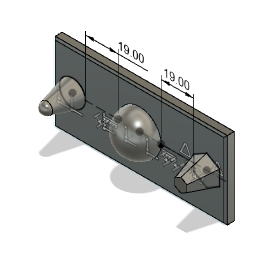
Tormach Milling Test (Autodesk Fusion 360 design; units mm, degrees)
Autodesk Fusion 360 part; units mm, degrees
note: some values were not read from the file. Set by a fixed rule: which sketch regions a step uses.
sketch "Sketch1" plane through (0, 0, 0) normal (0, 0, 1) x (1, 0, 0)
  line L0 (-50, 22.5) -> (50, 22.5)
  line L1 (50, 22.5) -> (50, -22.5)
  line L2 (50, -22.5) -> (-50, -22.5)
  line L3 (-50, -22.5) -> (-50, 22.5)
  line L4 (-50, 22.5) -> (50, -22.5) construction
  dimension "d1" = 100
  dimension "d2" = 45
  constraint horizontal L0
  constraint vertical L1
  constraint horizontal L2
  constraint vertical L3
  constraint midpoint origin L4
  measures "d1" distance of L0.start L0.end
  measures "d2" distance of L0.end L1.end
extrude "Extrude1" add sketch "Sketch1" along normal blind 5
sphere "SpherePrimitive1" add diameter 25 placed x (1, 0, 0) y (0, 1, 0) z (0, 0, 1) at (0, 0, 5)
box "BoxPrimitive1" cut length 45 width 100 height 15 placed x (0, 1, 0) y (1, 0, 0) z (0, 0, -1) at (-50, -22.5, 0)
sketch "Sketch5" plane through (0, 0, 5) normal (0, 0, 1) x (1, 0, 0)
  circle A0 centre (0, 0) radius 12.5
  line L0 (-50, -22.5) -> (50, -22.5)
  line L1 (50, -22.5) -> (50, 22.5)
  line L2 (50, 22.5) -> (-50, 22.5)
  line L3 (-50, 22.5) -> (-50, -22.5)
  line L4 (39, -8.6603) -> (46.5, -4.3301)
  line L5 (46.5, -4.3301) -> (46.5, 4.3301)
  line L6 (46.5, 4.3301) -> (39, 8.6603)
  line L7 (39, 8.6603) -> (31.5, 4.3301)
  line L8 (31.5, 4.3301) -> (31.5, -4.3301)
  line L9 (31.5, -4.3301) -> (39, -8.6603)
  line L10 (12.5, 0) -> (31.5, 0) construction
  line L11 (0, 0) -> (50, 0) construction
  line L12 (-12.5, 0) -> (-31.5, 0) construction
  circle A1 centre (-39, 0) radius 7.5
  point P0 (39, 0)
  dimension "d16" = 19
  dimension "d17" = 15
  dimension "d18" = 19
  dimension "d19" = 15
  constraint coincident A0 L10.start
  constraint midpoint L8 L10.end
  constraint horizontal L10
  constraint coincident A0.centre L11.start
  constraint midpoint L1 L11.end
  constraint collinear L10 L11
  constraint perpendicular L8 L10
  constraint coincident A0 L12.start
  constraint horizontal L12
  constraint collinear L11 L12
  constraint coincident L12 A1.centre
  constraint coincident L12.end A1
  measures "d16" distance of L10.start L10.end
  measures "d17" distance of L5 L8
  measures "d18" distance of L12.start L12.end
  measures "d19" diameter of A1
extrude "Extrude3" add sketch "Sketch5" along normal blind 15 draft -15 contours L4 L5 L6 L7 L8 L9 | A1
sketch "Sketch9" plane through (0, 0, 20) normal (0, 0, 1) x (1, 0, 0)
  circle A0 centre (-39, 0) radius 3.4808
  line L0 (-39, 3.4808) -> (-39, -3.4808)
  point P0 (-39, 0)
  constraint coincident A0 L0.start
  constraint coincident A0 L0.end
  constraint vertical L0
  constraint coincident L0 P0
revolve "Revolve1" add sketch "Sketch9" angle 180 about axis through (-39, 3.4808, 20) along (0, -1, 0) contours A0 L0 picked at (-38.2402, 0.8769)
chamfer "Chamfer1" distance 1 angle 45 4 edges at (0, -22.5, 5) (50, 0, 5) (0, 22.5, 5) (-50, 0, 5)
